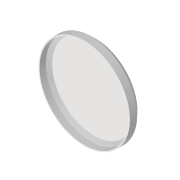
# Autodesk Inventor part: 00_Lid_Bonne_Mamman
Saved by Autodesk Inventor 2022 (Build 260153000, 153)
## iProperties
Created: 2022-10-10
Part Number: 00_Lid_Bonne_Mamman
Material: Generisch
Document SubType Name: Modeling
Designer: UC2
Density: 1 g/cm^3
Appearance: Vorgabe
Author: UC2
Autodesk Inventor part; units mm, degrees
ref_plane "YZ Plane" through (0, 0, 0) normal (1, 0, 0) x (0, 1, 0)
ref_plane "XZ Plane" through (0, 0, 0) normal (0, 1, 0) x (-1, 0, 0)
ref_plane "XY Plane" through (0, 0, 0) normal (0, 0, 1) x (1, 0, 0)
sketch "Skizze1" plane through (0, 0, 0) normal (0, 1, 0) x (-1, 0, 0)
  line L0 (0, 0) -> (-34.25, 0)
  line L1 (-34.25, 0) -> (-34.25, -1)
  line L2 (-34.25, -1) -> (-40.25, -1)
  line L3 (-40.25, -1) -> (-40.25, 0)
  line L4 (-40.25, 0) -> (-43.501, 3.052)
  line L5 (-43.501, 3.052) -> (-43.501, 10)
  line L6 (0, 0) -> (0, 1)
  line L7 (0, 1) -> (-39.3112, 1)
  line L8 (-39.3112, 1) -> (-42.501, 3.9945)
  line L9 (-42.501, 3.9945) -> (-42.501, 10)
  line L10 (-42.501, 10) -> (-43.501, 10)
  dimension "d0" = 34.25
  dimension "d1" = 1
  dimension "d2" = 6
  dimension "d3" = 10
  dimension "d4" = 1
  dimension "d5" = 1
  constraints: 22 end point, 4 perpendicular, 3 parallel, 2 vertical, 1 horizontal
  measures "d0" distance of L0.start L0.end
  measures "d1" distance of L0.end L1.end
  measures "d2" distance of L1.end L2.end
  measures "d3" distance from line of L5.end L0
  measures "d4" distance of L0.start L6.end
  measures "d5" distance between parallel lines of L9 L5
revolve "Umdrehung1" add sketch "Skizze1" angle 360 about axis through (0, 0, 0) along (0, 0, 1)
fillet "Rundung1" radius 1 6 edges at (-34.25, 0, 0) (-34.25, 0, -1) (-40.25, 0, -1) (-40.25, 0, 0) (-43.501, 0, 3.052) (-39.3112, 0, 1)
sketch "Skizze2" plane through (0, 0, 0) normal (0, 0, -1) x (-1, 0, 0)
  circle A0 centre (0.0031, -0.0027) radius 3 projected
  arc A1 (-12.0467, -11.77) -> (-7.3029, -12.5022) centre (-9.4998, -11.0022) ccw projected
  circle A2 centre (0.0031, -0.0027) radius 6
  circle A3 centre (-9.4998, -11.0022) radius 6
  line L0 (0.0031, -0.0027) -> (-9.4998, -11.0022)
  line L1 (-5.781, -6.2859) -> (-4.1232, -4.3669)
  line L2 (-4.1232, -4.3669) -> (-3.7157, -4.719)
  line L3 (-3.7157, -4.719) -> (-5.3735, -6.6379)
  line L4 (-5.3735, -6.6379) -> (-5.781, -6.2859)
  line L5 (-5.781, -6.2859) -> (-3.7157, -4.719) construction
  line L6 (-4.1232, -4.3669) -> (-5.3735, -6.6379) construction
  point P0 (0, 0)
  point P1 (-4.7484, -5.5024)
  point P2 (-5.5773, -6.4619)
  point P3 (-3.9194, -4.543)
  dimension "d8" = 12
  dimension "d9" = 12
  constraints: 14 end point, 3 midpoint, 2 centre point, 2 coincident, 2 parallel, 1 perpendicular
  measures "d8" diameter of A2
  measures "d9" diameter of A3
extrude "Extrusion1" cut sketch "Skizze2" against normal blind 10 contours A0 | A2 | A3 | L2 L3 L4 L0 | L0 L4 L1 L2
ref_plane "Arbeitsebene1" through (3.9194, -4.543, 0) normal (-0.7567077, -0.6537534, 0) x (0, 0, 1)
